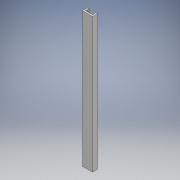
# Autodesk Inventor part: Barrière
Saved by Autodesk Inventor 2017 (Build 210142000, 142)
## iProperties
Part Number: Barrière
Material: Générique
Document SubType Name: Modeling
Designer: Geoff
Density: 1 g/cm^3
Appearance: Par défaut
Author: Geoff
Autodesk Inventor part; units mm, degrees
ref_plane "YZ Plane" through (0, 0, 0) normal (1, 0, 0) x (0, 1, 0)
ref_plane "XZ Plane" through (0, 0, 0) normal (0, 1, 0) x (-1, 0, 0)
ref_plane "XY Plane" through (0, 0, 0) normal (0, 0, 1) x (1, 0, 0)
sketch "Esquisse1" plane through (0, 0, 0) normal (1, 0, 0) x (0, 1, 0)
  line L0 (0, 0) -> (5, 0)
  line L1 (5, 0) -> (5, -30)
  line L2 (5, -30) -> (0, -30)
  line L3 (0, -30) -> (0, 0)
  dimension "d0" = 5
  dimension "d1" = 30
  constraints: 8 end point, 2 parallel, 1 horizontal, 1 perpendicular
  measures "d0" distance of L1.end L2.end
  measures "d1" distance of L0.end L1.end
extrude "Extrusion1" add sketch "Esquisse1" along normal blind 10
sketch "Esquisse2" plane through (0, 5, 0) normal (0, 1, 0) x (1, 0, 0)
  line L0 (0, 0) -> (5, 0)
  line L1 (0, 0) -> (10, 0) projected
  line L2 (5, 0) -> (5, 8)
  arc A0 (1.4921, 8.545) -> (8.5079, 8.545) centre (5, 8) ccw
  line L3 (5, 21.75) -> (5, 20.05)
  arc A1 (6.6798, 20.311) -> (3.3202, 20.311) centre (5, 20.05) ccw
  line L4 (1.4921, 8.545) -> (3.3202, 20.311)
  line L5 (8.5079, 8.545) -> (6.6798, 20.311)
  line L6 (5, 4.45) -> (5, 11.55)
  line L7 (5, 18.35) -> (5, 21.75)
  dimension "d4" = 8
  dimension "d5" = 7.1
  dimension "d6" = 17.3
  dimension "d7" = 1.7
  constraints: 14 end point, 7 point on circle, 2 centre point, 2 coincident, 2 midpoint, 2 tangent, 1 perpendicular, 1 point on line
  measures "d4" distance of L0.end L2.end
  measures "d5" diameter of A0
  measures "d6" distance of L6.start L3.start
  measures "d7" distance of L3.start L3.end
extrude "Extrusion2" cut sketch "Esquisse2" against normal blind 3.5
sketch "Esquisse3" plane through (0, 5, 0) normal (0, 1, 0) x (1, 0, 0)
  arc A0 (1.4921, 8.545) -> (8.5079, 8.545) centre (5, 8) ccw projected
  arc A1 (8.4161, 9.1358) -> (1.5839, 9.1358) centre (5, 8) ccw
  arc A2 (6.6798, 20.311) -> (3.3202, 20.311) centre (5, 20.05) ccw projected
  arc A3 (6.6798, 20.311) -> (3.3202, 20.311) centre (5, 20.05) ccw
  line L0 (1.4921, 8.545) -> (3.3202, 20.311) projected
  line L1 (3.3202, 20.311) -> (1.4921, 8.545)
  line L2 (6.6798, 20.311) -> (8.5079, 8.545)
  point P0 (0, 0)
  dimension "d24" = 7.2
  constraints: 4 end point, 4 point on circle, 3 tangent, 2 centre point, 2 coincident, 2 point on line, 1 collinear
  measures "d24" diameter of A1
extrude "Extrusion5" add sketch "Esquisse3" against normal blind 1.4 contours L0 A2 L2 A1
sketch "Esquisse5" plane through (0, 5, 0) normal (0, 1, 0) x (1, 0, 0)
  arc A0 (1.4921, 8.545) -> (8.5079, 8.545) centre (5, 8) ccw projected
  line L0 (5, 0) -> (1.45, 0)
  line L1 (0, 0) -> (10, 0) projected
  line L2 (1.45, 0) -> (1.45, 8)
  line L3 (1.45, 8) -> (8.55, 8)
  line L4 (8.55, 8) -> (8.55, 0)
  line L5 (8.55, 0) -> (1.45, 0)
  line L6 (5, 8) -> (5, 0)
  dimension "d27" = 3.55
  dimension "d28" = 7.1
  constraints: 12 end point, 4 perpendicular, 2 point on line, 1 vertical
  measures "d27" distance of L0.start L0.end
  measures "d28" distance of L2.end L3.end
extrude "Extrusion6" cut sketch "Esquisse5" against normal blind 3.5
sketch "Esquisse6" plane through (0, 5, 0) normal (0, 1, 0) x (1, 0, 0)
  arc A0 (8.4161, 9.1358) -> (1.5839, 9.1358) centre (5, 8) ccw projected
  line L0 (5, 8) -> (5, 0)
  line L1 (5, 0) -> (1.55, 0)
  line L2 (0, 0) -> (10, 0) projected
  line L3 (1.55, 0) -> (1.55, 6.5)
  line L4 (8.45, 6.5) -> (8.45, 0)
  line L5 (8.45, 0) -> (1.55, 0)
  line L6 (8.55, 8) -> (8.55, 0) projected
  line L7 (8.45, 6.5) -> (8.55, 6.5)
  line L8 (8.55, 6.5) -> (8.55, 0)
  line L9 (8.55, 0) -> (8.45, 0)
  line L10 (8.45, 0) -> (8.45, 6.5)
  line L11 (1.45, 0) -> (1.45, 8) projected
  line L12 (1.55, 6.5) -> (1.45, 6.5)
  line L13 (1.45, 6.5) -> (1.45, 0)
  line L14 (1.45, 0) -> (1.55, 0)
  line L15 (1.55, 0) -> (1.55, 6.5)
  dimension "d31" = 3.45
  dimension "d32" = 6.5
  dimension "d33" = 6.9
  dimension "d34" = 6.5
  constraints: 26 end point, 4 parallel, 4 perpendicular, 2 horizontal, 2 point on line, 1 vertical
  measures "d31" distance of L0.end L1.end
  measures "d32" distance of L1.end L3.end
  measures "d33" distance of L3.end L4.start
  measures "d34" distance of L4.start L4.end
extrude "Extrusion8" add sketch "Esquisse6" against normal blind 1.5
sketch "Esquisse7" plane through (0, 0, -30) normal (0, -1, 0) x (1, 0, 0)
  line L0 (0, 0) -> (10, 0)
  line L1 (10, 0) -> (10, -105)
  line L2 (10, -105) -> (0, -105)
  line L3 (0, -105) -> (0, 0)
  point P0 (0, 30)
  dimension "d39" = 10
  dimension "d40" = 105
  constraints: 8 end point, 2 parallel, 1 horizontal, 1 perpendicular
  measures "d39" distance of L1.end L2.end
  measures "d40" distance of L0.end L1.end
extrude "Extrusion9" add sketch "Esquisse7" against normal blind 5
